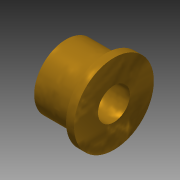
# Autodesk Inventor part: Sinterbuchse 35 60 325 48106
Saved by Autodesk Inventor 2014 (Build 180170000, 170)
## iProperties
Created: 2013-09-03
Part Number: Sinterbuchse 35 60 325 48106
Material: Allgemein
Document SubType Name: Modeling
Designer: vogel
Density: 1 g/cm^3
Appearance: Schweißnaht - Messing
Author: vogel
Autodesk Inventor part; units mm, degrees
ref_plane "YZ Plane" through (0, 0, 0) normal (1, 0, 0) x (0, 1, 0)
ref_plane "XZ Plane" through (0, 0, 0) normal (0, 1, 0) x (-1, 0, 0)
ref_plane "XY Plane" through (0, 0, 0) normal (0, 0, 1) x (1, 0, 0)
sketch "Skizze1" plane through (0, 0, 0) normal (0, 0, 1) x (1, 0, 0)
  line L0 (-7.2, 0) -> (1.2, 0) projected
  line L1 (0, -1) -> (0, 6) projected
  line L2 (-6, 2) -> (0, 2)
  line L3 (-1, 4) -> (-6, 4)
  line L4 (-6, 4) -> (-6, 2)
  line L5 (0, 2) -> (0, 5)
  line L6 (0, 5) -> (-1, 5)
  line L7 (-1, 5) -> (-1, 4)
  point P0 (0, 0)
  dimension "d0" = 4
  dimension "d1" = 8
  dimension "d2" = 10
  dimension "d3" = 1
  dimension "d4" = 6
  constraints: 12 end point, 3 parallel, 1 collinear, 1 horizontal, 1 point on line
  measures "d0" diameter of L2 L0
  measures "d1" diameter of L3 L0
  measures "d2" diameter of L6 L0
  measures "d3" distance of L5.end L6.end
  measures "d4" distance between parallel lines of L4 L1
revolve "Umdrehung1" add sketch "Skizze1" angle 360 about axis through (-10, 0, 0) along (1, 0, 0)
